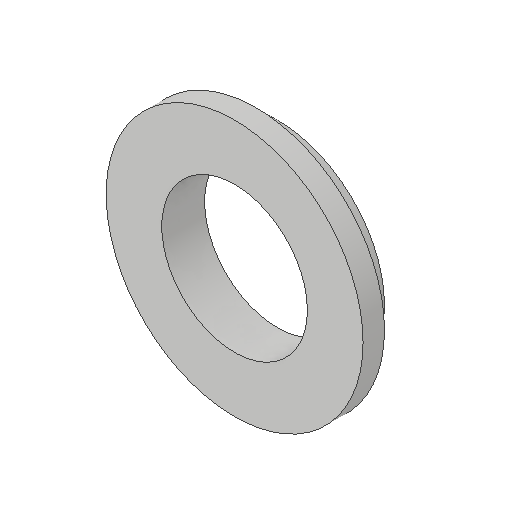
# Autodesk Inventor part: 3DP_PLA_Y_axis_drive_shaft_pulley_washer
Saved by Autodesk Inventor 2025 (Build 290162010, 162A)
## iProperties
Created: 2018-06-17
Part Number: 3DP_PLA_Y_axis_drive_shaft_pulley_washer
Material: Generic
Document SubType Name: Modeling
Designer: Andrzej
Density: 1 g/cm^3
Appearance: Default
Author: Andrzej
Autodesk Inventor part; units mm, degrees
ref_plane "YZ Plane" through (0, 0, 0) normal (1, 0, 0) x (0, 1, 0)
ref_plane "XZ Plane" through (0, 0, 0) normal (0, 1, 0) x (-1, 0, 0)
ref_plane "XY Plane" through (0, 0, 0) normal (0, 0, 1) x (1, 0, 0)
sketch "Sketch1" plane through (0, 0, 0) normal (0, 0, 1) x (1, 0, 0)
  circle A0 centre (0, 0) radius 4.5
  circle A1 centre (0, 0) radius 2.55
  dimension "d0" = 9
  dimension "d1" = 5.1
  constraints: 2 centre point, 2 coincident
  measures "d0" diameter of A0
  measures "d1" diameter of A1
extrude "Extrusion1" add sketch "Sketch1" along normal blind 1.5
chamfer "Chamfer1" distance 0.75 angle 45 1 edges at (-4.5, 0, 0)
body "Solid1"
